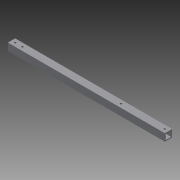
# Autodesk Inventor part: mounting block medium
Saved by Autodesk Inventor 2015 SP1 (Build 190203100, 203)
## iProperties
Created: 2015-01-17
Part Number: mounting block medium
Material: Generic
Document SubType Name: Modeling
Designer: Jarod
Density: 1 g/cm^3
Appearance: Default
Author: Jarod
Autodesk Inventor part; units mm, degrees
ref_plane "YZ Plane" through (0, 0, 0) normal (1, 0, 0) x (0, 1, 0)
ref_plane "XZ Plane" through (0, 0, 0) normal (0, 1, 0) x (-1, 0, 0)
ref_plane "XY Plane" through (0, 0, 0) normal (0, 0, 1) x (1, 0, 0)
sketch "Sketch1" plane through (0, 0, 0) normal (1, 0, 0) x (0, 1, 0)
  line L0 (0, 0) -> (25.4, 0)
  line L1 (25.4, 0) -> (25.4, -25.4)
  line L2 (25.4, -25.4) -> (0, -25.4)
  line L3 (0, -25.4) -> (0, 0)
  line L4 (3.175, -3.175) -> (22.225, -3.175)
  line L5 (22.225, -3.175) -> (22.225, -22.225)
  line L6 (22.225, -22.225) -> (3.175, -22.225)
  line L7 (3.175, -22.225) -> (3.175, -3.175)
  dimension "d0" = 25.4
  dimension "d1" = 25.4
  dimension "d2" = 19.05
  dimension "d3" = 19.05
  dimension "d4" = 3.175
  dimension "d5" = 3.175
  constraints: 16 end point, 4 parallel, 2 horizontal, 2 perpendicular
  measures "d0" distance of L1.end L2.end
  measures "d1" distance of L0.end L1.end
  measures "d2" distance of L5.end L6.end
  measures "d3" distance of L4.end L5.end
  measures "d4" distance between parallel lines of L3 L7
  measures "d5" distance between parallel lines of L0 L4
extrude "Extrusion1" add sketch "Sketch1" along normal blind 546.1
sketch "Sketch2" plane through (0, 25.4, 0) normal (0, 1, 0) x (1, 0, 0)
  line L0 (0, 0) -> (0, 25.4) projected
  line L1 (0, 0) -> (546.1, 0) projected
  line L2 (546.1, 25.4) -> (546.1, 0) projected
  line L3 (0, 25.4) -> (546.1, 25.4) projected
  point P0 (12.7, 12.7)
  point P1 (533.4, 12.7)
  dimension "d8" = 12.7
  dimension "d9" = 12.7
  dimension "d10" = 12.7
  dimension "d11" = 12.7
  measures "d8" distance from line of L1 point (12.7, 12.7)
  measures "d9" distance from line of point (12.7, 12.7) L0
  measures "d10" distance from line of L2 point (533.4, 12.7)
  measures "d11" distance from line of L1 point (533.4, 12.7)
hole "Hole1" at (12.7, 25.4, -12.7) at (533.4, 25.4, -12.7) direction (0, -1, 0) diameter 6.35 end through all
sketch "Sketch3" plane through (0, 25.4, 0) normal (0, 1, 0) x (1, 0, 0)
  circle A0 centre (12.7, 12.7) radius 3.175 projected
  circle A1 centre (533.4, 12.7) radius 3.175 projected
  line L0 (0, 0) -> (0, 25.4) projected
  line L1 (0, 0) -> (546.1, 0) projected
  line L2 (546.1, 25.4) -> (546.1, 0) projected
  line L3 (0, 25.4) -> (546.1, 25.4) projected
  point P0 (38.1, 12.7)
  point P1 (381, 12.7)
  dimension "d19" = 165.1
  dimension "d20" = 38.1
  dimension "d21" = 12.7
  dimension "d22" = 12.7
  measures "d19" distance from line of L2 point (381, 12.7)
  measures "d20" distance from line of L0 point (38.1, 12.7)
  measures "d21" distance from line of L1 point (38.1, 12.7)
  measures "d22" distance from line of L1 point (381, 12.7)
hole "Hole2" at (38.1, 25.4, -12.7) at (381, 25.4, -12.7) direction (0, -1, 0) diameter 6.35 end through all
body "Solid1"
